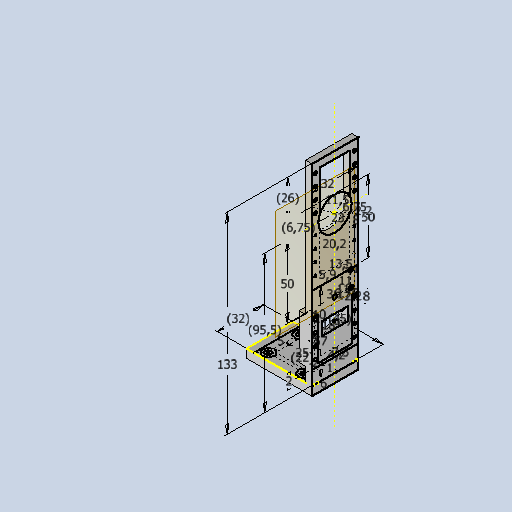
# Autodesk Inventor part: Support AX 12A haut
Saved by Autodesk Inventor 2022 (Build 260153000, 153)
## iProperties
Created: 2022-01-08
Part Number: Support AX 12A haut
Material: Générique
Document SubType Name: Modeling
Designer: victo
Density: 1 g/cm^3
Appearance: Par défaut
Source: UnKnown
Author: victo
Autodesk Inventor part; units mm, degrees
ref_plane "YZ Plane" through (0, 0, 0) normal (1, 0, 0) x (0, 1, 0)
ref_plane "XZ Plane" through (0, 0, 0) normal (0, 1, 0) x (-1, 0, 0)
ref_plane "Plan de construction4" through (0, 0, 21) normal (0, 0, 1) x (1, 0, 0)
sketch "Esquisse" plane through (0, 0, 21) normal (0, 0, 1) x (1, 0, 0)
  circle A0 centre (0, 0) radius 11.5
  line L0 (16, -11.5) -> (-16, -11.5) construction
  line L1 (-16, -11.5) -> (-16, 38.5)
  line L2 (-16, 38.5) -> (16, 38.5) construction
  line L3 (16, 38.5) -> (16, -11.5)
  line L4 (0, 0) -> (-13.5, 6.75) construction
  circle A1 centre (-13.5, 6.75) radius 1.1 construction
  line L5 (-13.5, 6.75) -> (-13.5, 14.75) construction
  line L6 (-13.5, 14.75) -> (-13.5, 22.75) construction
  line L7 (-13.5, 22.75) -> (-13.5, 30.75) construction
  circle A2 centre (-13.5, 30.75) radius 1.1 construction
  circle A3 centre (-13.5, 22.75) radius 1.1 construction
  circle A4 centre (-13.5, 14.75) radius 1.1 construction
  line L8 (-23.9117, 0) -> (22.6519, 0) construction
  line L9 (10.1, 32.6) -> (10.1, 5.4991) construction
  line L10 (-10.1, 5.4991) -> (-10.1, 32.6) construction
  line L11 (-10.1, 32.6) -> (10.1, 32.6) construction
  line L12 (16, -11.5) -> (0, 0) construction
  line L13 (-16, -11.5) -> (0, 0) construction
  line L14 (10.1, 5.4991) -> (-10.1, 5.4991) construction
  line L15 (16, 38.5) -> (-16, 38.5)
  line L16 (-16, 38.5) -> (-16, 95.5)
  line L17 (-16, 95.5) -> (16, 95.5)
  line L18 (16, 95.5) -> (16, 38.5)
  line L19 (0, -65.3) -> (0, 129.3) construction
  circle A5 centre (13.5, 6.75) radius 1.1 construction
  circle A6 centre (13.5, 30.75) radius 1.1 construction
  circle A7 centre (13.5, 22.75) radius 1.1 construction
  circle A8 centre (13.5, 14.75) radius 1.1 construction
  line L20 (-16, -11.5) -> (16, -11.5) construction
  line L21 (16, -11.5) -> (16, -37.5)
  line L22 (16, -37.5) -> (-16, -37.5)
  line L23 (-16, -37.5) -> (-16, -11.5)
  line L24 (16, 95.5) -> (-16, 95.5)
  line L25 (-16, 95.5) -> (-16, 101.5)
  line L26 (-16, 101.5) -> (16, 101.5)
  line L27 (16, 101.5) -> (16, 95.5)
  line L28 (16, -37.5) -> (-17.2597, -37.5)
  circle A9 centre (-13.5, -6.75) radius 1.1
  circle A10 centre (-13.5, -30.75) radius 1.1
  circle A11 centre (-13.5, -22.75) radius 1.1
  circle A12 centre (-13.5, -14.75) radius 1.1
  line L29 (10.1, -32.6) -> (10.1, -5.4991)
  line L30 (-10.1, -5.4991) -> (-10.1, -32.6)
  line L31 (-10.1, -32.6) -> (10.1, -32.6)
  circle A13 centre (13.5, -6.75) radius 1.1
  circle A14 centre (13.5, -14.75) radius 1.1
  circle A15 centre (13.5, -22.75) radius 1.1
  circle A16 centre (13.5, -30.75) radius 1.1
  line L32 (10.1, -32.6) -> (10.1, -5.4991)
  line L33 (-10.1, -5.4991) -> (-10.1, -32.6)
  line L34 (-10.1, -32.6) -> (10.1, -32.6)
  circle A17 centre (0, 50) radius 1.55
  circle A18 centre (-13.5, 56.75) radius 1.1
  circle A19 centre (-13.5, 64.75) radius 1.1
  circle A20 centre (-13.5, 72.75) radius 1.1
  circle A21 centre (-13.5, 80.75) radius 1.1
  circle A22 centre (13.5, 56.75) radius 1.1
  circle A23 centre (13.5, 64.75) radius 1.1
  circle A24 centre (13.5, 80.75) radius 1.1
  circle A25 centre (13.5, 72.75) radius 1.1
  line L35 (-13.5, 56.75) -> (-13.5, 64.75) construction
  line L36 (-13.5, 72.75) -> (-13.5, 64.75) construction
  line L37 (-13.5, 80.75) -> (-13.5, 72.75) construction
  line L38 (-13.5, 30.75) -> (-13.5, 56.75) construction
  line L39 (13.5, 56.75) -> (13.5, 64.75) construction
  line L40 (13.5, 64.75) -> (13.5, 72.75) construction
  line L41 (13.5, 72.75) -> (13.5, 80.75) construction
  line L42 (-13.5, 80.75) -> (13.5, 80.75) construction
  line L43 (-9, 69) -> (9, 69)
  line L44 (9, 69) -> (9, 60)
  line L45 (9, 60) -> (-9, 60)
  line L46 (-9, 60) -> (-9, 69)
  line L47 (-9, 69) -> (9, 60) construction
  line L48 (9, 69) -> (-9, 60) construction
  line L49 (16, 54.75) -> (11.5, 54.75)
  line L50 (11.5, 54.75) -> (11.5, 83.85)
  line L51 (11.5, 83.85) -> (-11.5, 83.85)
  line L52 (-11.5, 83.85) -> (-11.5, 54.75)
  line L53 (-11.5, 54.75) -> (-16, 54.75)
  line L54 (16, 85.85) -> (-16, 85.85)
  line L55 (0, 50) -> (-11, 50) construction
  line L56 (-11, 50) -> (-11, 39) construction
  circle A26 centre (-11, 50) radius 1.55
  circle A27 centre (-11, 39) radius 1.55
  point P0 (0, -11.5)
  point P1 (16, -11.5)
  point P2 (10.1, -5.4991)
  point P3 (0, 64.5)
  dimension "d107" = 23
  dimension "d133" = 6.75
  dimension "d135" = 2.2
  dimension "d137" = 8
  dimension "d138" = 20.2
  dimension "d160" = 50
  dimension "d161" = 5.9
  dimension "d162" = 32
  dimension "d163" = 11.5
  dimension "d169" = 26
  dimension "d224" = 57
  dimension "d225" = 6
  dimension "d240" = 13.5
  dimension "d247" = 95.5
  dimension "d248" = 133
  dimension "d249" = 50
  dimension "d250" = 3.1
  dimension "d254" = 6.75
  dimension "d255" = 8
  dimension "d256" = 2.2
  dimension "d257" = 6.75
  dimension "d258" = 10
  dimension "d259" = 9
  dimension "d260" = 18
  dimension "d261" = 2
  dimension "d262" = 2
  dimension "d263" = 2
  dimension "d264" = 2
  dimension "d267" = 3.1
  dimension "d268" = 11
  dimension "d269" = 11
  constraints: 110 end point, 28 centre point, 23 equal length, 16 symmetric about line, 11 equal radius, 11 point on line, 10 horizontal, 10 perpendicular, 7 coincident, 6 vertical, 3 collinear, 2 midpoint, 2 point on circle, 12 other
  measures "d107" diameter of A0
  measures "d133" vertical distance of L4.start L4.end
  measures "d135" diameter of A1
  measures "d137" distance of L5.start L5.end
  measures "d138" distance between parallel lines of L10 L9
  measures "d160" distance between parallel lines of L2 L0
  measures "d161" distance between parallel lines of L2 L11
  measures "d162" distance between parallel lines of L3 L1
  measures "d163" distance from line of L0 point (0, 0)
  measures "d169" distance between parallel lines of L22 L0
  measures "d224" distance between parallel lines of L17 L2
  measures "d225" distance between parallel lines of L26 L17
  measures "d240" distance from line of L19 L5.end
  measures "d247" distance from line of L17 point (0, 0)
  measures "d248" distance between parallel lines of L17 L28
  measures "d249" distance of L55.start point (0, 0)
  measures "d250" diameter of A17
  measures "d254" vertical distance of L4.start A13.centre
  measures "d255" distance of L35.start L35.end
  measures "d256" diameter of A18
  measures "d257" vertical distance of L35.start L55.start
  measures "d258" distance from line of L45 L55.start
  measures "d259" distance between parallel lines of L43 L45
  measures "d260" distance between parallel lines of L46 L44
  measures "d261" distance from line of L50 L39.start
  measures "d262" distance from line of L49 L39.start
  measures "d263" distance between parallel lines of L54 L51
  measures "d264" distance edge to line of A24 L51
  measures "d267" diameter of A27
  measures "d268" distance of L55.start L55.end
  measures "d269" distance of L55.end L56.end
extrude "Face fixation moteur" add sketch "Esquisse" against normal blind 4 contours L1 L15 A27 L3 L21 L22 L23 | L16 L53 L52 L51 L50 L49 L18 L15 A27 | L16 L54 L18 L49 L50 L51 L52 L53 | L16 L17 L18 L54
extrude "Creux moteur" [suppressed]
extrude "Rai basl" add sketch "Esquisse" against normal blind 45 contours L25 L26 L27 L17
sketch "Esquisse16" plane through (-16, 95.5, 17) normal (0, -1, 0) x (1, 0, 0)
  line L0 (0, 0) -> (0, -41) projected
  line L1 (32, -41) -> (0, -41) projected
  line L2 (32, 0) -> (32, -41) projected
  line L3 (5, -6) -> (27, -6) construction
  line L4 (27, -6) -> (27, -31) construction
  line L5 (27, -31) -> (5, -31) construction
  line L6 (5, -31) -> (5, -6) construction
  line L7 (0, 0) -> (0, -41) projected
  line L8 (0, -1) -> (5, -6) construction
  line L9 (5, -31) -> (0, -36) construction
  line L10 (0, -41) -> (32, -41) projected
  line L11 (27, -31) -> (32, -36) construction
  circle A0 centre (5, -6) radius 2.1
  circle A1 centre (27, -6) radius 2.1
  circle A2 centre (27, -31) radius 2.1
  circle A3 centre (5, -31) radius 2.1
  line L12 (6.1207, -10.1826) -> (1.9381, -9.0619)
  line L13 (1.9381, -9.0619) -> (0.8174, -4.8793)
  line L14 (0.8174, -4.8793) -> (3.8793, -1.8174)
  line L15 (3.8793, -1.8174) -> (8.0619, -2.9381)
  line L16 (8.0619, -2.9381) -> (9.1826, -7.1207)
  line L17 (9.1826, -7.1207) -> (6.1207, -10.1826)
  line L18 (9.1826, -29.8793) -> (8.0619, -34.0619)
  line L19 (8.0619, -34.0619) -> (3.8793, -35.1826)
  line L20 (3.8793, -35.1826) -> (0.8174, -32.1207)
  line L21 (0.8174, -32.1207) -> (1.9381, -27.9381)
  line L22 (1.9381, -27.9381) -> (6.1207, -26.8174)
  line L23 (6.1207, -26.8174) -> (9.1826, -29.8793)
  line L24 (25.8793, -26.8174) -> (30.0619, -27.9381)
  line L25 (30.0619, -27.9381) -> (31.1826, -32.1207)
  line L26 (31.1826, -32.1207) -> (28.1207, -35.1826)
  line L27 (28.1207, -35.1826) -> (23.9381, -34.0619)
  line L28 (23.9381, -34.0619) -> (22.8174, -29.8793)
  line L29 (22.8174, -29.8793) -> (25.8793, -26.8174)
  line L30 (22.8174, -7.1207) -> (23.9381, -2.9381)
  line L31 (23.9381, -2.9381) -> (28.1207, -1.8174)
  line L32 (28.1207, -1.8174) -> (31.1826, -4.8793)
  line L33 (31.1826, -4.8793) -> (30.0619, -9.0619)
  line L34 (30.0619, -9.0619) -> (25.8793, -10.1826)
  line L35 (25.8793, -10.1826) -> (22.8174, -7.1207)
  line L36 (7.6517, -8.6517) -> (24.3483, -8.6517) construction
  line L37 (24.3483, -8.6517) -> (24.3483, -28.3483) construction
  line L38 (24.3483, -28.3483) -> (7.6517, -28.3483) construction
  line L39 (7.6517, -28.3483) -> (7.6517, -8.6517) construction
  line L40 (32, 4) -> (0, 4) projected
  line L41 (32, 0) -> (32, -41) projected
  line L42 (0, 0) -> (0, -41) projected
  line L43 (0, 4) -> (32, 4) projected
  line L44 (0, -1) -> (32, -1)
  line L45 (32, -1) -> (27, -6) construction
  line L46 (0, 0) -> (32, 0) projected
  line L47 (32, -36) -> (0, -36)
  point P0 (16, -17)
  point P1 (28.4, 4)
  point P2 (30.6, 4)
  point P3 (28.4, 4)
  point P4 (30.6, 4)
  point P5 (1.4, 4)
  point P6 (3.6, 4)
  point P7 (1.4, 4)
  point P8 (3.6, 4)
  point P9 (1.4, 4)
  point P10 (3.6, 4)
  point P11 (1.4, 4)
  point P12 (3.6, 4)
  point P13 (28.4, 4)
  point P14 (30.6, 4)
  point P15 (28.4, 4)
  point P16 (30.6, 4)
  dimension "d228" = 5
  dimension "d230" = 4.2
  dimension "d231" = 7.5
  dimension "d232" = 25
  dimension "d233" = 22
  dimension "d245" = 45
  dimension "d246" = 32
  dimension "d251" = 1
  dimension "d253" = 5
  constraints: 76 end point, 8 coincident, 8 point on line, 7 perpendicular, 4 centre point, 4 midpoint, 4 parallel, 3 equal radius, 2 horizontal, 52 other
  measures "d228" distance between parallel lines of L0 L6
  measures "d230" diameter of A0
  measures "d231" distance between parallel lines of L17 L14
  measures "d232" distance between parallel lines of L5 L3
  measures "d233" distance between parallel lines of L6 L4
  measures "d245" distance from line of L10 L43.start
  measures "d246" distance of L0.end L1.start
  measures "d251" distance between parallel lines of L46 L44
  measures "d253" distance between parallel lines of L47 L5
extrude "Extrusion23" cut sketch "Esquisse16" against normal through all contours A0 | A1 | A2 | A3
extrude "Extrusion25" add sketch "Esquisse" against normal blind 8.5 contours L16 L54 L18 L49 L50 L51 L52 L53
